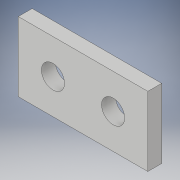
# Autodesk Inventor part: attache
Saved by Autodesk Inventor 2017 (Build 210142000, 142)
## iProperties
Created: 2017-03-09
Part Number: attache
Material: Generic
Document SubType Name: Modeling
Designer: LaFaucheuse
Density: 1 g/cm^3
Appearance: Default
Author: LaFaucheuse
Autodesk Inventor part; units mm, degrees
ref_plane "YZ Plane" through (0, 0, 0) normal (1, 0, 0) x (0, 1, 0)
ref_plane "XZ Plane" through (0, 0, 0) normal (0, 1, 0) x (-1, 0, 0)
ref_plane "XY Plane" through (0, 0, 0) normal (0, 0, 1) x (1, 0, 0)
sketch "Esquisse1" plane through (0, 0, 0) normal (0, 0, 1) x (1, 0, 0)
  line L0 (0, 0) -> (28, 0)
  line L1 (28, 0) -> (28, 15)
  line L2 (28, 15) -> (0, 15)
  line L3 (0, 15) -> (0, 0)
  circle A0 centre (7.5, 7.5) radius 2.5
  circle A1 centre (20.5, 7.5) radius 2.5
  dimension "d0" = 28
  dimension "d1" = 15
  dimension "d3" = 5
  dimension "d4" = 5
  dimension "d5" = 7.5
  dimension "d6" = 7.5
  dimension "d7" = 7.5
  dimension "d8" = 7.5
  constraints: 8 end point, 2 centre point, 2 parallel, 1 horizontal, 1 perpendicular
  measures "d0" distance of L1.end L2.end
  measures "d1" distance of L0.end L1.end
  measures "d3" diameter of A1
  measures "d4" diameter of A0
  measures "d5" distance from line of L1 A1.centre
  measures "d6" distance from line of L2 A1.centre
  measures "d7" distance from line of L3 A0.centre
  measures "d8" distance from line of L2 A0.centre
extrude "Extrusion1" add sketch "Esquisse1" along normal blind 3
